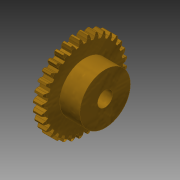
# Autodesk Inventor part: Zahnrad Messing z32
Saved by Autodesk Inventor 2019.3 (Build 233278000, 278)
## iProperties
Category: PARTsolutions
Company: MAEDLER
Created: 2018-08-20
Part Number: Zahnrad Messing z32
Material: Messing, weicher Gelbton, geschweißt
Catalog Web Link: www.cadenas.de
Description: Stzr Messing Ms58-Spur Gears, Brass, Helical Tooth Right Hand, with one-sided hub
Vendor: MAEDLER
Document SubType Name: Modeling
Designer: psadmin
Manufacturer: MAEDLER
Mass: 5.6 g
Surface Area: 7.4577 cm^2
Volume: 0.667925 cm^3
Density: 8.38417 g/cm^3
Appearance: Schweißnaht - Messing
PSOL_IDENT_0: {$CADENAS_DATA\23d-libs\maedler\antriebselemente\stirnzahnraeder\stirnzahnraeder_messing\stzr_messin
PSOL_IDENT_1: g_ms58.prj},204 {VTYP=3D},{NB=Stzr Messing Ms58 26103200},{LINA=Stzr Messing Ms58 26103200},{NN=Stzr
PSOL_IDENT_2: Messing Ms58},{DATE=03.08.2018 09:08:56},{GEOMDATE=26.07.2018 09:15:44},{VERSION=},{LINEID=370},{WB
PSOL_IDENT_3: VAR=},{WBNUMERIC=}  {NB=Stzr Messing Ms58 26103200},{LINA=Stzr Messing Ms58 26103200},{KT=DUMMY},{AR
PSOL_IDENT_4: TNR=26103200},{WST=Messing (Ms58)},{M=0.5},{Z=32},{PDF=PDF Katalogseite},{B1=2.0},{DA=17.00},{D=16.0
PSOL_IDENT_5: 0},{NL=4},{ND=10},{B=3.00},{MD=3.5},{GEW=5.600}
NN: Stzr Messing Ms58
NT: Spur Gears, Brass, Helical Tooth Right Hand, with one-sided hub
NB: Stzr Messing Ms58 26103200
NBSYN: Stzr Messing Ms58 $ARTNR.
LINA: Stzr Messing Ms58 26103200
ARTNR: 26103200
WST: Messing (Ms58)
M: 0.5
Z: 32
PDF: PDF Katalogseite
B1: 2
DA: 17
D: 16
NL: 4
ND: 10
B: 3
MD: 3.5
GEW: 5.6
SUPPLIER: MAEDLER
ARTICLENO: Stzr Messing Ms58 26103200
BOMINFO: Stzr Messing Ms58 26103200
CREATOR: CADENAS GmbH
Title: Stzr Messing Ms58 26103200
Author: Cadenas PARTsolutions
Comments: Spur Gears, Brass, Helical Tooth Right Hand, with one-sided hub
Autodesk Inventor part; units mm, degrees
ref_plane "YZ Plane" through (0, 0, 0) normal (1, 0, 0) x (0, 1, 0)
ref_plane "XZ Plane" through (0, 0, 0) normal (0, 1, 0) x (-1, 0, 0)
ref_plane "XY Plane" through (0, 0, 0) normal (0, 0, 1) x (1, 0, 0)
sketch "Skizze_1" plane through (0, 0, 0) normal (0, 0, 1) x (1, 0, 0)
  line L0 (6, 0) -> (0, 0)
  line L1 (0, 1.5) -> (6, 1.5)
  line L2 (6, 1.5) -> (6, 5)
  line L3 (6, 5) -> (2, 5)
  line L4 (2, 5) -> (2, 8)
  line L5 (2, 8) -> (1, 10.7475)
  line L6 (1, 10.7475) -> (0, 8)
  line L7 (0, 8) -> (0, 1.5)
  constraints: 16 end point
revolve "Revolution1" add sketch "Skizze_1" angle 360 about axis through (6, 0, 0) along (1, 0, 0)
sketch "Skizze_2" plane through (2, 0, 0) normal (1, 0, 0) x (0, 0, -1)
  circle A0 centre (0, 0) radius 25.5
  arc A1 (-8.4738, -0.6671) -> (-8.4411, -0.9988) centre (0, 0) ccw
  line L0 (-8.4411, -0.9988) -> (-7.9181, -1.1419)
  line L1 (-7.9181, -1.1419) -> (-7.3998, -1.2217)
  arc A2 (-7.3998, -1.2217) -> (-7.3041, -1.7031) centre (0, 0) ccw
  line L2 (-7.3041, -1.7031) -> (-7.7524, -1.9751)
  line L3 (-7.7524, -1.9751) -> (-8.1808, -2.3075)
  arc A3 (-8.1808, -2.3075) -> (-8.084, -2.6264) centre (0, 0) ccw
  line L4 (-8.084, -2.6264) -> (-7.5432, -2.6647)
  line L5 (-7.5432, -2.6647) -> (-7.0193, -2.6419)
  arc A4 (-7.0193, -2.6419) -> (-6.8315, -3.0953) centre (0, 0) ccw
  line L6 (-6.8315, -3.0953) -> (-7.2181, -3.4496)
  line L7 (-7.2181, -3.4496) -> (-7.5735, -3.8591)
  arc A5 (-7.5735, -3.8591) -> (-7.4163, -4.1531) centre (0, 0) ccw
  line L8 (-7.4163, -4.1531) -> (-6.8783, -4.0851)
  line L9 (-6.8783, -4.0851) -> (-6.369, -3.9605)
  arc A6 (-6.369, -3.9605) -> (-6.0964, -4.3686) centre (0, 0) ccw
  line L10 (-6.0964, -4.3686) -> (-6.4064, -4.7914)
  line L11 (-6.4064, -4.7914) -> (-6.6751, -5.2625)
  arc A7 (-6.6751, -5.2625) -> (-6.4636, -5.5201) centre (0, 0) ccw
  line L12 (-6.4636, -5.5201) -> (-5.9492, -5.3485)
  line L13 (-5.9492, -5.3485) -> (-5.474, -5.1269)
  arc A8 (-5.474, -5.1269) -> (-5.1269, -5.474) centre (0, 0) ccw
  line L14 (-5.1269, -5.474) -> (-5.3485, -5.9492)
  line L15 (-5.3485, -5.9492) -> (-5.5201, -6.4636)
  arc A9 (-5.5201, -6.4636) -> (-5.2625, -6.6751) centre (0, 0) ccw
  line L16 (-5.2625, -6.6751) -> (-4.7914, -6.4064)
  line L17 (-4.7914, -6.4064) -> (-4.3686, -6.0964)
  arc A10 (-4.3686, -6.0964) -> (-3.9605, -6.369) centre (0, 0) ccw
  line L18 (-3.9605, -6.369) -> (-4.0851, -6.8783)
  line L19 (-4.0851, -6.8783) -> (-4.1531, -7.4163)
  arc A11 (-4.1531, -7.4163) -> (-3.8591, -7.5735) centre (0, 0) ccw
  line L20 (-3.8591, -7.5735) -> (-3.4496, -7.2181)
  line L21 (-3.4496, -7.2181) -> (-3.0953, -6.8315)
  arc A12 (-3.0953, -6.8315) -> (-2.6419, -7.0193) centre (0, 0) ccw
  line L22 (-2.6419, -7.0193) -> (-2.6647, -7.5432)
  line L23 (-2.6647, -7.5432) -> (-2.6264, -8.084)
  arc A13 (-2.6264, -8.084) -> (-2.3075, -8.1808) centre (0, 0) ccw
  line L24 (-2.3075, -8.1808) -> (-1.9751, -7.7524)
  line L25 (-1.9751, -7.7524) -> (-1.7031, -7.3041)
  arc A14 (-1.7031, -7.3041) -> (-1.2217, -7.3998) centre (0, 0) ccw
  line L26 (-1.2217, -7.3998) -> (-1.1419, -7.9181)
  line L27 (-1.1419, -7.9181) -> (-0.9988, -8.4411)
  arc A15 (-0.9988, -8.4411) -> (-0.6671, -8.4738) centre (0, 0) ccw
  line L28 (-0.6671, -8.4738) -> (-0.4247, -7.9887)
  line L29 (-0.4247, -7.9887) -> (-0.2454, -7.496)
  arc A16 (-0.2454, -7.496) -> (0.2454, -7.496) centre (0, 0) ccw
  line L30 (0.2454, -7.496) -> (0.4247, -7.9887)
  line L31 (0.4247, -7.9887) -> (0.6671, -8.4738)
  arc A17 (0.6671, -8.4738) -> (0.9988, -8.4411) centre (0, 0) ccw
  line L32 (0.9988, -8.4411) -> (1.1419, -7.9181)
  line L33 (1.1419, -7.9181) -> (1.2217, -7.3998)
  arc A18 (1.2217, -7.3998) -> (1.7031, -7.3041) centre (0, 0) ccw
  line L34 (1.7031, -7.3041) -> (1.9751, -7.7524)
  line L35 (1.9751, -7.7524) -> (2.3075, -8.1808)
  arc A19 (2.3075, -8.1808) -> (2.6264, -8.084) centre (0, 0) ccw
  line L36 (2.6264, -8.084) -> (2.6647, -7.5432)
  line L37 (2.6647, -7.5432) -> (2.6419, -7.0193)
  arc A20 (2.6419, -7.0193) -> (3.0953, -6.8315) centre (0, 0) ccw
  line L38 (3.0953, -6.8315) -> (3.4496, -7.2181)
  line L39 (3.4496, -7.2181) -> (3.8591, -7.5735)
  arc A21 (3.8591, -7.5735) -> (4.1531, -7.4163) centre (0, 0) ccw
  line L40 (4.1531, -7.4163) -> (4.0851, -6.8783)
  line L41 (4.0851, -6.8783) -> (3.9605, -6.369)
  arc A22 (3.9605, -6.369) -> (4.3686, -6.0964) centre (0, 0) ccw
  line L42 (4.3686, -6.0964) -> (4.7914, -6.4064)
  line L43 (4.7914, -6.4064) -> (5.2625, -6.6751)
  arc A23 (5.2625, -6.6751) -> (5.5201, -6.4636) centre (0, 0) ccw
  line L44 (5.5201, -6.4636) -> (5.3485, -5.9492)
  line L45 (5.3485, -5.9492) -> (5.1269, -5.474)
  arc A24 (5.1269, -5.474) -> (5.474, -5.1269) centre (0, 0) ccw
  line L46 (5.474, -5.1269) -> (5.9492, -5.3485)
  line L47 (5.9492, -5.3485) -> (6.4636, -5.5201)
  arc A25 (6.4636, -5.5201) -> (6.6751, -5.2625) centre (0, 0) ccw
  line L48 (6.6751, -5.2625) -> (6.4064, -4.7914)
  line L49 (6.4064, -4.7914) -> (6.0964, -4.3686)
  arc A26 (6.0964, -4.3686) -> (6.369, -3.9605) centre (0, 0) ccw
  line L50 (6.369, -3.9605) -> (6.8783, -4.0851)
  line L51 (6.8783, -4.0851) -> (7.4163, -4.1531)
  arc A27 (7.4163, -4.1531) -> (7.5735, -3.8591) centre (0, 0) ccw
  line L52 (7.5735, -3.8591) -> (7.2181, -3.4496)
  line L53 (7.2181, -3.4496) -> (6.8315, -3.0953)
  arc A28 (6.8315, -3.0953) -> (7.0193, -2.6419) centre (0, 0) ccw
  line L54 (7.0193, -2.6419) -> (7.5432, -2.6647)
  line L55 (7.5432, -2.6647) -> (8.084, -2.6264)
  arc A29 (8.084, -2.6264) -> (8.1808, -2.3075) centre (0, 0) ccw
  line L56 (8.1808, -2.3075) -> (7.7524, -1.9751)
  line L57 (7.7524, -1.9751) -> (7.3041, -1.7031)
  arc A30 (7.3041, -1.7031) -> (7.3998, -1.2217) centre (0, 0) ccw
  line L58 (7.3998, -1.2217) -> (7.9181, -1.1419)
  line L59 (7.9181, -1.1419) -> (8.4411, -0.9988)
  arc A31 (8.4411, -0.9988) -> (8.4738, -0.6671) centre (0, 0) ccw
  line L60 (8.4738, -0.6671) -> (7.9887, -0.4247)
  line L61 (7.9887, -0.4247) -> (7.496, -0.2454)
  arc A32 (7.496, -0.2454) -> (7.496, 0.2454) centre (0, 0) ccw
  line L62 (7.496, 0.2454) -> (7.9887, 0.4247)
  line L63 (7.9887, 0.4247) -> (8.4738, 0.6671)
  arc A33 (8.4738, 0.6671) -> (8.4411, 0.9988) centre (0, 0) ccw
  line L64 (8.4411, 0.9988) -> (7.9181, 1.1419)
  line L65 (7.9181, 1.1419) -> (7.3998, 1.2217)
  arc A34 (7.3998, 1.2217) -> (7.3041, 1.7031) centre (0, 0) ccw
  line L66 (7.3041, 1.7031) -> (7.7524, 1.9751)
  line L67 (7.7524, 1.9751) -> (8.1808, 2.3075)
  arc A35 (8.1808, 2.3075) -> (8.084, 2.6264) centre (0, 0) ccw
  line L68 (8.084, 2.6264) -> (7.5432, 2.6647)
  line L69 (7.5432, 2.6647) -> (7.0193, 2.6419)
  arc A36 (7.0193, 2.6419) -> (6.8315, 3.0953) centre (0, 0) ccw
  line L70 (6.8315, 3.0953) -> (7.2181, 3.4496)
  line L71 (7.2181, 3.4496) -> (7.5735, 3.8591)
  arc A37 (7.5735, 3.8591) -> (7.4163, 4.1531) centre (0, 0) ccw
  line L72 (7.4163, 4.1531) -> (6.8783, 4.0851)
  line L73 (6.8783, 4.0851) -> (6.369, 3.9605)
  arc A38 (6.369, 3.9605) -> (6.0964, 4.3686) centre (0, 0) ccw
  line L74 (6.0964, 4.3686) -> (6.4064, 4.7914)
  line L75 (6.4064, 4.7914) -> (6.6751, 5.2625)
  arc A39 (6.6751, 5.2625) -> (6.4636, 5.5201) centre (0, 0) ccw
  line L76 (6.4636, 5.5201) -> (5.9492, 5.3485)
  line L77 (5.9492, 5.3485) -> (5.474, 5.1269)
  arc A40 (5.474, 5.1269) -> (5.1269, 5.474) centre (0, 0) ccw
  line L78 (5.1269, 5.474) -> (5.3485, 5.9492)
  line L79 (5.3485, 5.9492) -> (5.5201, 6.4636)
  arc A41 (5.5201, 6.4636) -> (5.2625, 6.6751) centre (0, 0) ccw
  line L80 (5.2625, 6.6751) -> (4.7914, 6.4064)
  line L81 (4.7914, 6.4064) -> (4.3686, 6.0964)
  arc A42 (4.3686, 6.0964) -> (3.9605, 6.369) centre (0, 0) ccw
  line L82 (3.9605, 6.369) -> (4.0851, 6.8783)
  line L83 (4.0851, 6.8783) -> (4.1531, 7.4163)
  arc A43 (4.1531, 7.4163) -> (3.8591, 7.5735) centre (0, 0) ccw
  line L84 (3.8591, 7.5735) -> (3.4496, 7.2181)
  line L85 (3.4496, 7.2181) -> (3.0953, 6.8315)
  arc A44 (3.0953, 6.8315) -> (2.6419, 7.0193) centre (0, 0) ccw
  line L86 (2.6419, 7.0193) -> (2.6647, 7.5432)
  line L87 (2.6647, 7.5432) -> (2.6264, 8.084)
  arc A45 (2.6264, 8.084) -> (2.3075, 8.1808) centre (0, 0) ccw
  line L88 (2.3075, 8.1808) -> (1.9751, 7.7524)
  line L89 (1.9751, 7.7524) -> (1.7031, 7.3041)
  arc A46 (1.7031, 7.3041) -> (1.2217, 7.3998) centre (0, 0) ccw
  line L90 (1.2217, 7.3998) -> (1.1419, 7.9181)
  line L91 (1.1419, 7.9181) -> (0.9988, 8.4411)
  arc A47 (0.9988, 8.4411) -> (0.6671, 8.4738) centre (0, 0) ccw
  line L92 (0.6671, 8.4738) -> (0.4247, 7.9887)
  line L93 (0.4247, 7.9887) -> (0.2454, 7.496)
  arc A48 (0.2454, 7.496) -> (-0.2454, 7.496) centre (0, 0) ccw
  line L94 (-0.2454, 7.496) -> (-0.4247, 7.9887)
  line L95 (-0.4247, 7.9887) -> (-0.6671, 8.4738)
  arc A49 (-0.6671, 8.4738) -> (-0.9988, 8.4411) centre (0, 0) ccw
  line L96 (-0.9988, 8.4411) -> (-1.1419, 7.9181)
  line L97 (-1.1419, 7.9181) -> (-1.2217, 7.3998)
  arc A50 (-1.2217, 7.3998) -> (-1.7031, 7.3041) centre (0, 0) ccw
  line L98 (-1.7031, 7.3041) -> (-1.9751, 7.7524)
  line L99 (-1.9751, 7.7524) -> (-2.3075, 8.1808)
  arc A51 (-2.3075, 8.1808) -> (-2.6264, 8.084) centre (0, 0) ccw
  line L100 (-2.6264, 8.084) -> (-2.6647, 7.5432)
  line L101 (-2.6647, 7.5432) -> (-2.6419, 7.0193)
  arc A52 (-2.6419, 7.0193) -> (-3.0953, 6.8315) centre (0, 0) ccw
  line L102 (-3.0953, 6.8315) -> (-3.4496, 7.2181)
  line L103 (-3.4496, 7.2181) -> (-3.8591, 7.5735)
  arc A53 (-3.8591, 7.5735) -> (-4.1531, 7.4163) centre (0, 0) ccw
  line L104 (-4.1531, 7.4163) -> (-4.0851, 6.8783)
  line L105 (-4.0851, 6.8783) -> (-3.9605, 6.369)
  arc A54 (-3.9605, 6.369) -> (-4.3686, 6.0964) centre (0, 0) ccw
  line L106 (-4.3686, 6.0964) -> (-4.7914, 6.4064)
  line L107 (-4.7914, 6.4064) -> (-5.2625, 6.6751)
  arc A55 (-5.2625, 6.6751) -> (-5.5201, 6.4636) centre (0, 0) ccw
  line L108 (-5.5201, 6.4636) -> (-5.3485, 5.9492)
  line L109 (-5.3485, 5.9492) -> (-5.1269, 5.474)
  arc A56 (-5.1269, 5.474) -> (-5.474, 5.1269) centre (0, 0) ccw
  line L110 (-5.474, 5.1269) -> (-5.9492, 5.3485)
  line L111 (-5.9492, 5.3485) -> (-6.4636, 5.5201)
  arc A57 (-6.4636, 5.5201) -> (-6.6751, 5.2625) centre (0, 0) ccw
  line L112 (-6.6751, 5.2625) -> (-6.4064, 4.7914)
  line L113 (-6.4064, 4.7914) -> (-6.0964, 4.3686)
  arc A58 (-6.0964, 4.3686) -> (-6.369, 3.9605) centre (0, 0) ccw
  line L114 (-6.369, 3.9605) -> (-6.8783, 4.0851)
  line L115 (-6.8783, 4.0851) -> (-7.4163, 4.1531)
  arc A59 (-7.4163, 4.1531) -> (-7.5735, 3.8591) centre (0, 0) ccw
  line L116 (-7.5735, 3.8591) -> (-7.2181, 3.4496)
  line L117 (-7.2181, 3.4496) -> (-6.8315, 3.0953)
  arc A60 (-6.8315, 3.0953) -> (-7.0193, 2.6419) centre (0, 0) ccw
  line L118 (-7.0193, 2.6419) -> (-7.5432, 2.6647)
  line L119 (-7.5432, 2.6647) -> (-8.084, 2.6264)
  arc A61 (-8.084, 2.6264) -> (-8.1808, 2.3075) centre (0, 0) ccw
  line L120 (-8.1808, 2.3075) -> (-7.7524, 1.9751)
  line L121 (-7.7524, 1.9751) -> (-7.3041, 1.7031)
  arc A62 (-7.3041, 1.7031) -> (-7.3998, 1.2217) centre (0, 0) ccw
  line L122 (-7.3998, 1.2217) -> (-7.9181, 1.1419)
  line L123 (-7.9181, 1.1419) -> (-8.4411, 0.9988)
  arc A63 (-8.4411, 0.9988) -> (-8.4738, 0.6671) centre (0, 0) ccw
  line L124 (-8.4738, 0.6671) -> (-7.9887, 0.4247)
  line L125 (-7.9887, 0.4247) -> (-7.496, 0.2454)
  arc A64 (-7.496, 0.2454) -> (-7.496, -0.2454) centre (0, 0) ccw
  line L126 (-7.496, -0.2454) -> (-7.9887, -0.4247)
  line L127 (-7.9887, -0.4247) -> (-8.4738, -0.6671)
  constraints: 256 end point, 128 point on circle, 65 centre point
extrude "Extrusion1" cut sketch "Skizze_2" along normal mid plane 12
body "Solid1"
